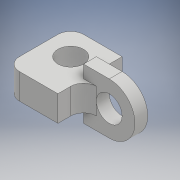
# Autodesk Inventor part: 22
Saved by Autodesk Inventor 2017 (Build 210142000, 142)
## iProperties
Part Number: 22
Material: 一般
Document SubType Name: Modeling
Designer: Brian
Density: 1 g/cm^3
Appearance: 預設
Author: Brian
Autodesk Inventor part; units mm, degrees
ref_plane "YZ Plane" through (0, 0, 0) normal (1, 0, 0) x (0, 1, 0)
ref_plane "XZ Plane" through (0, 0, 0) normal (0, 1, 0) x (-1, 0, 0)
ref_plane "XY Plane" through (0, 0, 0) normal (0, 0, 1) x (1, 0, 0)
sketch "草圖1" plane through (0, 0, 0) normal (0, 0, 1) x (1, 0, 0)
  line L0 (0, 30) -> (-40, 30)
  line L1 (-40, 30) -> (-40, -20)
  line L2 (-40, -20) -> (0, -20)
  line L3 (0, -20) -> (0, 30)
  point P0 (0, 0)
  dimension "d0" = 40
  dimension "d1" = 20
  dimension "d2" = 50
  constraints: 8 end point, 2 parallel, 1 horizontal, 1 perpendicular, 1 point on line
  measures "d0" distance of L1.end L2.end
  measures "d1" distance from line of L2 point (0, 0)
  measures "d2" distance of L0.end L1.end
extrude "擠出1" add sketch "草圖1" along normal mid plane 20
sketch "草圖2" plane through (0, 0, 0) normal (0, 1, 0) x (-1, 0, 0)
  line L0 (0, -20) -> (-40, -20)
  line L1 (-40, -20) -> (-40, 20)
  line L2 (-40, 20) -> (0, 20)
  line L3 (0, 20) -> (0, -20)
  line L4 (40, -10) -> (0, -10) projected
  line L5 (0, 10) -> (0, -10) projected
  point P0 (0, 0)
  dimension "d5" = 40
  dimension "d6" = 40
  dimension "d7" = 10
  dimension "d8" = 0
  constraints: 8 end point, 2 parallel, 1 horizontal, 1 perpendicular
  measures "d5" distance of L2.end L0.start
  measures "d6" distance of L0.start L0.end
  measures "d7" distance between parallel lines of L4 L0
  measures "d8" distance between parallel lines of L5 L3
extrude "擠出2" add sketch "草圖2" along normal blind 10
fillet "圓角1" radius 10 2 edges at (0, 10, 0) (0, 0, 0)
fillet "圓角2" radius 20 2 edges at (40, 5, 20) (40, 5, -20)
hole "孔1" at (20, 10, 0) direction (0, -1, 0) diameter 20 depth 72000 tip angle 118
hole "孔2" at (-20, 10, -10) direction (0, 0, 1) diameter 20 depth 20 tip angle 118
fillet "圓角3" radius 10 2 edges at (-40, 30, 0) (-40, -20, 0)
